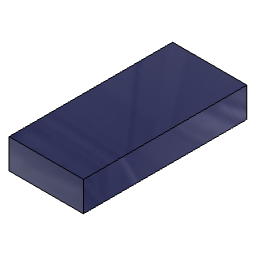
Boards v3 (Autodesk Fusion 360 design; units mm, degrees)
Autodesk Fusion 360 part; units mm, degrees
sketch "Sketch1" plane through (0, 0, 0) normal (0, 0, 1) x (1, 0, 0)
  line L0 (0, 0) -> (63.5, 0)
  line L1 (63.5, 0) -> (63.5, 139.7)
  line L2 (63.5, 139.7) -> (0, 139.7)
  line L3 (0, 139.7) -> (0, 0)
  dimension "d1" = 139.7
  dimension "d2" = 63.5
  constraint horizontal L0
  constraint vertical L1
  constraint horizontal L2
  constraint vertical L3
  constraint coincident L0.start L3.end
  measures "d1" distance of L0.start L2.end
  measures "d2" distance of L0.start L0.end
extrude "Extrude1" add sketch "Sketch1" along normal blind 25.4
sketch "Sketch2" plane through (0, 0, 0) normal (0, 0, 1) x (1, 0, 0)
  circle A0 centre (8, 16) radius 1.5875
  circle A1 centre (55.5, 16) radius 1.5875
  circle A2 centre (31.75, 66) radius 1.5875
  line L0 (63.5, 0) -> (63.5, 139.7)
  line L1 (0, 139.7) -> (0, 0)
  line L2 (0, 0) -> (63.5, 0)
  dimension "d5" = 3.175
  dimension "d6" = 3.175
  dimension "d7" = 3.175
  dimension "d9" = 8
  dimension "d10" = 8
  dimension "d11" = 16
  dimension "d12" = 16
  dimension "d13" = 66
  dimension "d14" = 31.75
  measures "d5" diameter of A0
  measures "d6" diameter of A1
  measures "d7" diameter of A2
  measures "d9" distance of A1.centre L0
  measures "d10" distance of A0.centre L1
  measures "d11" distance of A1.centre L2
  measures "d12" distance of A0.centre L2
  measures "d13" distance of A2.centre L2
  measures "d14" distance of A2.centre L0
extrude "Extrude2" cut sketch "Sketch2" along normal blind 10
